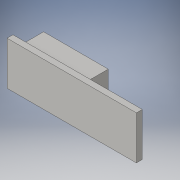
# Autodesk Inventor part: Track v3 Access Cover
Saved by Autodesk Inventor 2016 (Build 200138000, 138)
## iProperties
Created: 2016-05-24
Part Number: Track v3 Access Cover
Material: Generic
Document SubType Name: Modeling
Designer: xdlea
Density: 1 g/cm^3
Appearance: Default
Author: xdlea
Autodesk Inventor part; units mm, degrees
ref_plane "YZ Plane" through (0, 0, 0) normal (1, 0, 0) x (0, 1, 0)
ref_plane "XZ Plane" through (0, 0, 0) normal (0, 1, 0) x (-1, 0, 0)
ref_plane "XY Plane" through (0, 0, 0) normal (0, 0, 1) x (1, 0, 0)
sketch "Sketch1" plane through (0, 0, 0) normal (0, 0, 1) x (1, 0, 0)
  line L0 (-18.7642, -6.2928) -> (0, -6.2929)
  line L1 (18.7643, -6.2928) -> (18.7643, 6.2929)
  line L2 (18.7643, 6.2929) -> (0, 6.2928)
  line L3 (-18.7642, 6.2928) -> (-18.7642, 2.5971)
  line L4 (-18.7642, -6.2928) -> (18.7643, 6.2929) construction
  line L5 (18.7643, -6.2928) -> (-18.7642, 6.2928) construction
  line L6 (0, 6.2928) -> (0, 2.5972)
  line L7 (0, 6.2928) -> (-18.7642, 6.2928)
  line L8 (0, -6.2929) -> (18.7643, -6.2928)
  line L9 (0, 2.5972) -> (-18.7642, 2.5971)
  line L10 (0, 2.5972) -> (0, -6.2929)
  line L11 (-18.7642, 2.5971) -> (-18.7642, -6.2928)
  point P0 (0, 0)
  point P1 (0, 0)
  point P2 (0, 0)
  dimension "d0" = 12.5857
  dimension "d1" = 37.5285
  dimension "d5" = 8.89
  constraints: 24 end point, 6 parallel, 4 midpoint, 4 perpendicular, 2 horizontal, 2 point on line, 1 vertical alignment
  measures "d0" distance of L1.start L1.end
  measures "d1" distance of L1.end L3.start
  measures "d5" distance between parallel lines of L0 L9
extrude "Extrusion1" add sketch "Sketch1" along normal blind 1.7145
extrude "Extrusion2" add sketch "Sketch1" against normal blind 8.89 contours L11 L9 L10 L0
body "Solid1"
